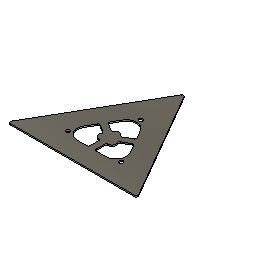
PCB (Autodesk Fusion 360 design; units mm, degrees)
Autodesk Fusion 360 part; units mm, degrees
sketch "Sketch1" plane through (0, 0, 0) normal (0, 0, 1) x (1, 0, 0)
  circle A0 centre (-190.0028, 38.6598) radius 2.5
  circle A1 centre (-223.4863, -19.3348) radius 2.5
  circle A2 centre (-156.5107, -19.3321) radius 2.5
  line L0 (-270.2459, -44.3327) -> (-191.7303, 91.6603)
  line L1 (-188.2662, 91.6603) -> (-109.7506, -44.3327)
  line L2 (-111.4826, -47.3327) -> (-268.5139, -47.3327)
  line L3 (-274.0245, -46.8774) -> (-272.6069, -49.3327)
  line L4 (-274.0245, -46.8774) -> (-191.4162, 96.2043)
  line L5 (-188.5801, 96.204) -> (-191.4221, 96.204)
  line L6 (-107.3967, -49.3327) -> (-105.9755, -46.8713)
  line L7 (-107.3967, -49.3327) -> (-272.6069, -49.3327)
  line L8 (-188.5801, 96.204) -> (-105.9755, -46.8713)
  arc A3 (-270.2459, -44.3327) -> (-268.5139, -47.3327) centre (-268.5139, -45.3327) ccw
  arc A4 (-188.2662, 91.6603) -> (-191.7303, 91.6603) centre (-189.9983, 90.6603) ccw
  arc A5 (-111.4826, -47.3327) -> (-109.7506, -44.3327) centre (-111.4826, -45.3327) ccw
  arc A6 (-219.1504, -3.8327) -> (-207.8921, -23.3327) centre (-207.8921, -10.3327) ccw
  arc A7 (-178.7399, 27.1603) -> (-201.2566, 27.1603) centre (-189.9983, 20.6603) ccw
  arc A8 (-172.1044, -23.3327) -> (-160.8461, -3.8327) centre (-172.1044, -10.3327) ccw
  arc A9 (-185.6681, 9.1603) -> (-194.3284, 9.1603) centre (-189.9983, 6.6603) ccw
  arc A10 (-200.0979, -0.8327) -> (-195.7678, -8.3327) centre (-195.7678, -3.3327) ccw
  arc A11 (-184.2287, -8.3327) -> (-179.8986, -0.8327) centre (-184.2287, -3.3327) ccw
  line L9 (-182.9361, 8.4283) -> (-173.4098, 13.9283)
  line L10 (-179.1666, 1.8993) -> (-169.6403, 7.3993)
  line L11 (-206.4769, 14.1788) -> (-197.0336, 8.5351)
  line L12 (-200.7511, 1.9755) -> (-210.1943, 7.6193)
  line L13 (-186.2287, -10.3327) -> (-186.2287, -21.3327)
  line L14 (-193.7678, -10.3327) -> (-193.7678, -21.3327)
  line L15 (-194.3284, 9.1603) -> (-194.2756, 9.2518)
  line L16 (-200.0451, -0.7412) -> (-200.0979, -0.8327)
  line L17 (-207.8921, -23.3327) -> (-195.7678, -23.3327)
  line L18 (-184.2287, -23.3327) -> (-172.1044, -23.3327)
  line L19 (-201.2566, 27.1603) -> (-207.1829, 16.8956)
  line L20 (-212.9524, 6.9025) -> (-219.1504, -3.8327)
  line L21 (-160.8461, -3.8327) -> (-166.9082, 6.6673)
  line L22 (-172.6777, 16.6603) -> (-178.7399, 27.1603)
  arc A12 (-185.6681, 9.1603) -> (-182.9361, 8.4283) centre (-183.9361, 10.1603) ccw
  arc A13 (-173.4098, 13.9283) -> (-172.6777, 16.6603) centre (-174.4098, 15.6603) ccw
  arc A14 (-166.9082, 6.6673) -> (-169.6403, 7.3993) centre (-168.6403, 5.6673) ccw
  arc A15 (-179.1666, 1.8993) -> (-179.8986, -0.8327) centre (-178.1666, 0.1673) ccw
  arc A16 (-184.2287, -8.3327) -> (-186.2287, -10.3327) centre (-184.2287, -10.3327) ccw
  arc A17 (-193.7678, -10.3327) -> (-195.7678, -8.3327) centre (-195.7678, -10.3327) ccw
  arc A18 (-200.0451, -0.7412) -> (-200.7511, 1.9755) centre (-201.7771, 0.2588) ccw
  arc A19 (-197.0336, 8.5351) -> (-194.2756, 9.2518) centre (-196.0076, 10.2518) ccw
  arc A20 (-207.1829, 16.8956) -> (-206.4769, 14.1788) centre (-205.4509, 15.8956) ccw
  arc A21 (-210.1943, 7.6193) -> (-212.9524, 6.9025) centre (-211.2204, 5.9025) ccw
  arc A22 (-195.7678, -23.3327) -> (-193.7678, -21.3327) centre (-195.7678, -21.3327) ccw
  arc A23 (-186.2287, -21.3327) -> (-184.2287, -23.3327) centre (-184.2287, -21.3327) ccw
  dimension "d1" = 5
  dimension "d2" = 5
  dimension "d3" = 5
  dimension "d5" = 120
  dimension "d11" = 2.842
  dimension "d12" = 120
  dimension "d13" = 60
  dimension "d16" = 120
  dimension "d17" = 120
  dimension "d18" = 120
  dimension "d19" = 2
  dimension "d20" = 2
  dimension "d21" = 2
  dimension "d22" = 2
  dimension "d23" = 60
  dimension "d24" = 60
  dimension "d25" = 24
  dimension "d26" = 24
  dimension "d27" = 24
  dimension "d28" = 13
  dimension "d32" = 5
  dimension "d34" = 2
  dimension "d35" = 2
  dimension "d36" = 2
  dimension "d37" = 2
  dimension "d38" = 2
  dimension "d39" = 2
  dimension "d40" = 2
  dimension "d41" = 2
  constraint horizontal L2
  constraint parallel L1 L8
  constraint tangent L2 A3
  constraint tangent L0 A3
  constraint tangent L0 A4
  constraint tangent L1 A4
  constraint equal A3 A4
  constraint tangent L1 A5
  constraint tangent L2 A5
  constraint equal A3 A5
  constraint horizontal L17
  constraint tangent A6 L19
  constraint tangent A6 L17
  constraint tangent A7 L19
  constraint tangent A7 L21
  constraint equal A6 A7
  constraint tangent A8 L17
  constraint tangent A8 L21
  constraint equal A6 A8
  constraint tangent A9 L15
  constraint tangent A10 L15
  constraint equal A9 A10
  constraint equal A9 A11
  constraint perpendicular L9 L21
  constraint perpendicular L10 L21
  constraint parallel L11 L12
  constraint perpendicular L13 L17
  constraint perpendicular L14 L17
  constraint collinear L15 L16
  constraint collinear L17 L18
  constraint collinear L19 L20
  constraint collinear L21 L22
  constraint tangent L9 A12
  constraint coincident A9.start A12.start
  constraint tangent L9 A13
  constraint tangent L22 A13
  constraint tangent L10 A14
  constraint tangent L21 A14
  constraint equal A13 A14
  constraint tangent L10 A15
  constraint equal A13 A15
  constraint coincident A11.end A15.end
  constraint tangent L13 A16
  constraint equal A13 A16
  constraint coincident A11.start A16.start
  constraint tangent L14 A17
  constraint equal A13 A17
  constraint coincident A10.end A17.end
  constraint tangent L12 A18
  constraint tangent L16 A18
  constraint equal A13 A18
  constraint tangent L11 A19
  constraint tangent L15 A19
  constraint equal A13 A19
  constraint tangent L11 A20
  constraint tangent L19 A20
  constraint equal A13 A20
  constraint tangent L12 A21
  constraint tangent L20 A21
  constraint equal A13 A21
  constraint tangent L14 A22
  constraint tangent L17 A22
  constraint equal A13 A22
  constraint tangent L13 A23
  constraint tangent L18 A23
  constraint equal A13 A23
  measures "d1" diameter of A0
  measures "d2" diameter of A2
  measures "d3" diameter of A1
  measures "d5" angle of L3 L4
  measures "d11" horizontal distance of L5.start L5.end
  measures "d12" angle of L4 L5
  measures "d13" angle of L0 L2
  measures "d16" angle of L3 L7
  measures "d17" angle of L6 L7
  measures "d18" angle of L6 L8
  measures "d19" distance of L1 L8
  measures "d20" distance of L0 L4
  measures "d21" distance of L2 L7
  measures "d22" radius of A3
  measures "d23" angle of L19 L21
  measures "d24" angle of L17 L21
  measures "d25" distance of L1 L21
  measures "d26" distance of L0 L19
  measures "d27" distance of L2 L17
  measures "d28" radius of A6
  measures "d32" radius of A9
  measures "d34" distance of A9.centre L9
  measures "d35" distance of A11.centre L10
  measures "d36" distance of A10.centre L12
  measures "d37" distance of A9.centre L11
  measures "d38" distance of A10.centre L14
  measures "d39" distance of A11.centre L13
  measures "d40" radius of A12
  measures "d41" radius of A13
extrude "Extrude1" add sketch "Sketch1" along normal blind 1.6 contours L0 L1 L2 A3 A4 A5
